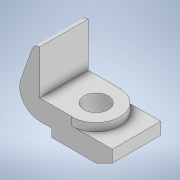
# Autodesk Inventor part: Assignment 1.7 - Hanger Jaw
Saved by Autodesk Inventor 2021.1 (Build 251245000, 245)
## iProperties
Created: 2021-05-14
Part Number: Assignment 1.7 - Hanger Jaw
Material: Generic
Document SubType Name: Modeling
Designer: as000166
Density: 1 g/cm^3
Appearance: Default
Author: as000166
Autodesk Inventor part; units mm, degrees
ref_plane "YZ Plane" through (0, 0, 0) normal (1, 0, 0) x (0, 1, 0)
ref_plane "XZ Plane" through (0, 0, 0) normal (0, 1, 0) x (-1, 0, 0)
ref_plane "XY Plane" through (0, 0, 0) normal (0, 0, 1) x (1, 0, 0)
sketch "Sketch1" plane through (0, 0, 0) normal (0, 0, 1) x (1, 0, 0)
  line L0 (0, 0) -> (69.85, 0)
  line L1 (0, 0) -> (0, 12.7)
  line L2 (95.25, 12.7) -> (69.85, 0)
  line L3 (0, 12.7) -> (-19.05, 12.7)
  line L4 (95.25, 31.75) -> (95.25, 12.7)
  line L5 (-19.05, 44.45) -> (31.75, 44.45)
  line L6 (31.75, 44.45) -> (31.75, 31.75)
  line L7 (31.75, 31.75) -> (95.25, 31.75)
  arc A0 (-48.5968, 56.0712) -> (-19.05, 12.7) centre (-19.05, 44.45) ccw
  line L8 (-19.05, 44.45) -> (-19.05, 95.25)
  line L9 (-19.05, 95.25) -> (-19.05, 101.6)
  arc A1 (-19.05, 114.3) -> (-31.2013, 105.2927) centre (-19.05, 101.6) ccw
  line L10 (-19.05, 101.6) -> (-19.05, 114.3)
  line L11 (-49.3376, 53.975) -> (-30.8232, 106.3625)
  dimension "d0" = 69.85
  dimension "d1" = 12.7
  dimension "d6" = 19.05
  dimension "d17" = 50.8
  dimension "d18" = 12.7
  dimension "d26" = 50.8
  dimension "d29" = 6.35
  dimension "d30" = 25.4
  constraints: 24 end point, 6 point on circle, 4 vertical, 3 horizontal, 2 centre point, 2 perpendicular, 2 point on line, 1 coincident
  measures "d0" distance of L0.start L0.end
  measures "d1" distance of L0.start L1.end
  measures "d6" distance of L3.end L1.end
  measures "d17" distance of L5.start L5.end
  measures "d18" distance of L5.end L6.end
  measures "d26" distance of L8.start L8.end
  measures "d29" distance of L8.end L9.end
  measures "d30" diameter of A1
extrude "Extrusion1" add sketch "Sketch1" against normal blind 76.2 contours L1 L3 A0 L11 A1 L10 L9 L8 L5 L6 L7 L4 L2 L0
sketch "Sketch3" plane through (-19.05, 44.45, 0) normal (0, 1, 0) x (1, 0, 0)
  arc A0 (50.8, -0.4913) -> (50.8, 75.7087) centre (50.8, 37.6087) ccw
  line L0 (50.8, 75.7087) -> (50.8, -0.4913)
  line L1 (50.8, 0) -> (50.8, 76.2) projected
  point P0 (19.05, 0)
  dimension "d40" = 76.2
  constraints: 2 end point, 2 point on circle, 1 centre point, 1 collinear, 1 point on line
  measures "d40" diameter of A0
extrude "Extrusion2" add sketch "Sketch3" against normal up to surface (12.7 mm away)
sketch "Sketch4" plane through (-19.05, 44.45, -76.2) normal (0, 1, 0) x (1, 0, 0)
  point P0 (19.05, -76.2)
  point P1 (50.9967, -38.2666)
hole "Hole2" at (31.9467, 44.45, -37.9334) direction (0, -1, 0) diameter 38.1 end through all
body "Solid1"
